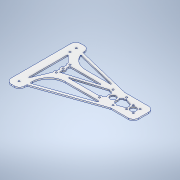
# Autodesk Inventor part: slidesthing
Saved by Autodesk Inventor 2020 (Build 240168000, 168)
## iProperties
Created: 2020-01-10
Part Number: slidesthing
Material: Aluminum 6061
Document SubType Name: Modeling
Designer: xj82b
Density: 2.7 g/cm^3
Appearance: Aluminum - Flat
Mass: 257.407 g
Surface Area: 278.616 cm^2
Volume: 36.001 cm^3
Author: xj82b
Autodesk Inventor part; units mm, degrees
ref_plane "YZ Plane" through (0, 0, 0) normal (1, 0, 0) x (0, 1, 0)
ref_plane "XZ Plane" through (0, 0, 0) normal (0, 1, 0) x (-1, 0, 0)
ref_plane "XY Plane" through (0, 0, 0) normal (0, 0, 1) x (1, 0, 0)
sketch "Sketch1" plane through (0, 0, 0) normal (0, 1, 0) x (-1, 0, 0)
  line L0 (0, 0) -> (0, -286.0722)
  line L1 (0, -286.0722) -> (-32, -286.0722)
  line L2 (-32, -286.0722) -> (-32, -238.0722)
  line L3 (-32, -238.0722) -> (-232, -238.0722)
  line L4 (-232, -238.0722) -> (-232, -190.0722)
  line L5 (-232, -190.0722) -> (-32, -190.0722)
  circle A0 centre (-16, -271.0722) radius 2
  circle A1 centre (-16, -256.0722) radius 2
  circle A2 centre (-16, -136.0722) radius 2
  circle A3 centre (-208, -214.0722) radius 7
  circle A4 centre (-160, -214.0722) radius 7
  circle A5 centre (-42, -230.0722) radius 2
  circle A6 centre (-144, -230.0722) radius 2
  circle A7 centre (-144, -198.0722) radius 2
  circle A8 centre (-176, -198.0722) radius 2
  circle A9 centre (-176, -230.0722) radius 2
  circle A10 centre (-200, -222.0722) radius 2
  circle A11 centre (-216, -222.0722) radius 2
  circle A12 centre (-216, -206.0722) radius 2
  circle A13 centre (-200, -206.0722) radius 2
  circle A14 centre (-42, -214.0722) radius 2
  line L6 (-32, -121.0722) -> (0, -121.0722)
  line L7 (-32, -190.0722) -> (-32, -121.0722)
  point P0 (-32, 0)
  point P1 (-16, -286.0722)
  point P2 (-232, -214.0722)
  dimension "d1" = 32
  dimension "d2" = 48
  dimension "d3" = 48
  dimension "d4" = 4
  dimension "d5" = 4
  dimension "d6" = 4
  dimension "d9" = 150
  dimension "d10" = 15
  dimension "d11" = 30
  dimension "d14" = 216
  dimension "d15" = 14
  dimension "d16" = 14
  dimension "d17" = 24
  dimension "d18" = 48
  dimension "d21" = 4
  dimension "d22" = 8
  dimension "d23" = 42
  dimension "d24" = 4
  dimension "d25" = 4
  dimension "d26" = 4
  dimension "d27" = 4
  dimension "d28" = 32
  dimension "d29" = 32
  dimension "d30" = 16
  dimension "d31" = 16
  dimension "d32" = 4
  dimension "d33" = 4
  dimension "d34" = 4
  dimension "d35" = 4
  dimension "d36" = 16
  dimension "d37" = 16
  dimension "d38" = 8
  dimension "d39" = 8
  dimension "d55" = 4
  dimension "d56" = 16
  dimension "d64" = 15
  dimension "d65" = 69
  constraints: 16 end point, 15 centre point, 7 vertical alignment, 6 horizontal alignment, 4 perpendicular, 3 point on line, 2 midpoint, 1 horizontal, 1 parallel, 1 vertical
  measures "d1" distance of L0.end L1.end
  measures "d2" distance of L1.end L2.end
  measures "d3" distance of L3.end L4.end
  measures "d4" diameter of A0
  measures "d5" diameter of A1
  measures "d6" diameter of A2
  measures "d9" distance from line of L1 A2.centre
  measures "d10" distance from line of L1 A0.centre
  measures "d11" distance from line of A1.centre L1
  measures "d14" distance from line of A1.centre L4
  measures "d15" diameter of A3
  measures "d16" diameter of A4
  measures "d17" distance from line of L4 A3.centre
  measures "d18" distance of A3.centre A4.centre
  measures "d21" diameter of A5
  measures "d22" distance from line of L3 A5.centre
  measures "d23" distance from line of L0 A5.centre
  measures "d24" diameter of A6
  measures "d25" diameter of A7
  measures "d26" diameter of A8
  measures "d27" diameter of A9
  measures "d28" distance of A9.centre A6.centre
  measures "d29" distance of A7.centre A6.centre
  measures "d30" horizontal distance of A4.centre A6.centre
  measures "d31" horizontal distance of A4.centre A6.centre
  measures "d32" diameter of A10
  measures "d33" diameter of A11
  measures "d34" diameter of A12
  measures "d35" diameter of A13
  measures "d36" distance of A11.centre A10.centre
  measures "d37" distance of A12.centre A11.centre
  measures "d38" horizontal distance of A3.centre A11.centre
  measures "d39" horizontal distance of A3.centre A11.centre
  measures "d55" diameter of A14
  measures "d56" distance of A14.centre A5.centre
  measures "d64" distance from line of A2.centre L6
  measures "d65" distance of L5.end L6.start
extrude "Extrusion1" add sketch "Sketch1" along normal blind 3.175
fillet "Fillet1" radius 12 6 edges at (232, 1.5875, -190.0722) (232, 1.5875, -238.0722) (32, 1.5875, -286.0722) (0, 1.5875, -286.0722) (32, 1.5875, -121.0722) (0, 1.5875, -121.0722)
fillet "Fillet2" radius 39 2 edges at (32, 1.5875, -190.0722) (32, 1.5875, -238.0722)
sketch "Sketch2" plane through (0, 3.175, 0) normal (0, 1, 0) x (1, 0, 0)
  circle A0 centre (16, 271.0722) radius 2 construction
  circle A1 centre (16, 271.0722) radius 3 construction
  circle A2 centre (16, 256.0722) radius 3 construction
  circle A3 centre (16, 256.0722) radius 2 construction
  circle A4 centre (42, 230.0722) radius 2 construction
  arc A5 (39.8787, 227.9509) -> (39.1086, 230.872) centre (42, 230.0722) ccw construction
  circle A6 centre (16, 136.0722) radius 2 construction
  circle A7 centre (16, 136.0722) radius 3 construction
  circle A8 centre (144, 230.0722) radius 2 construction
  circle A9 centre (144, 230.0722) radius 3 construction
  circle A10 centre (176, 230.0722) radius 2 construction
  circle A11 centre (176, 230.0722) radius 3 construction
  circle A12 centre (176, 198.0722) radius 2 construction
  circle A13 centre (176, 198.0722) radius 3 construction
  circle A14 centre (144, 198.0722) radius 2 construction
  circle A15 centre (144, 198.0722) radius 3 construction
  circle A16 centre (216, 222.0722) radius 2 construction
  circle A17 centre (216, 222.0722) radius 3 construction
  circle A18 centre (216, 206.0722) radius 2 construction
  circle A19 centre (216, 206.0722) radius 3 construction
  circle A20 centre (200, 206.0722) radius 2 construction
  circle A21 centre (200, 206.0722) radius 3 construction
  circle A22 centre (16, 136.0722) radius 2 construction
  circle A23 centre (176, 230.0722) radius 2 construction
  circle A24 centre (200, 222.0722) radius 3 construction
  circle A25 centre (200, 222.0722) radius 2 construction
  circle A26 centre (200, 206.0722) radius 2 construction
  circle A27 centre (216, 206.0722) radius 2 construction
  circle A28 centre (216, 222.0722) radius 2 construction
  line L0 (13, 136.0722) -> (13, 256.0722)
  line L1 (44.1213, 232.1935) -> (18.1213, 258.1935)
  line L2 (19, 256.0722) -> (19, 135.5292)
  line L3 (39.8787, 227.9509) -> (13.8787, 253.9509)
  circle A29 centre (16, 256.0722) radius 6
  circle A30 centre (42, 230.0722) radius 6
  circle A31 centre (16, 136.0722) radius 6
  circle A32 centre (42, 214.0722) radius 3 construction
  circle A33 centre (42, 214.0722) radius 2 construction
  circle A34 centre (42, 214.0722) radius 6
  line L4 (39, 214.0722) -> (39, 228.8296)
  line L5 (45, 213.5854) -> (45, 230.0722)
  line L6 (39.6062, 233.0722) -> (144, 233.0722)
  line L7 (147, 230.0722) -> (147, 198.0722)
  line L8 (141, 230.0722) -> (141, 198.0722)
  line L9 (144, 227.0722) -> (42, 227.0722)
  line L10 (143.5351, 195.1085) -> (41.5351, 211.1085)
  line L11 (42.4649, 217.036) -> (144.4649, 201.036)
  circle A35 centre (144, 230.0722) radius 6
  circle A36 centre (144, 198.0722) radius 6
  circle A37 centre (42, 198.0722) radius 2
  circle A38 centre (42, 198.0722) radius 3 construction
  circle A39 centre (42, 198.0722) radius 6
  line L12 (42, 201.0722) -> (144.2339, 201.0722)
  line L13 (42, 195.0722) -> (144, 195.0722)
  line L14 (45, 223.4471) -> (45, 216.6383)
  line L15 (45, 214.0722) -> (45, 198.0722)
  line L16 (39, 198.0722) -> (39, 223.6428)
  line L17 (13.2334, 137.2324) -> (39.2334, 199.2324)
  line L18 (18.7666, 134.912) -> (44.7666, 196.912)
  circle A40 centre (176, 230.0722) radius 6
  circle A41 centre (176, 198.0722) radius 2 projected
  circle A42 centre (176, 198.0722) radius 6
  circle A43 centre (200, 206.0722) radius 6
  circle A44 centre (200, 222.0722) radius 6
  circle A45 centre (216, 222.0722) radius 6
  circle A46 centre (216, 206.0722) radius 6
  line L19 (175.0513, 227.2262) -> (199.0513, 219.2262)
  line L20 (197, 222.0722) -> (197, 206.0722)
  line L21 (199.0513, 208.9183) -> (175.0513, 200.9183)
  line L22 (179, 230.0722) -> (179, 198.0722)
  circle A47 centre (3, 196.0722) radius 3 construction
  line L23 (0, 274.0722) -> (0, 133.0722) construction
  circle A48 centre (160, 214.0722) radius 3 construction
  circle A49 centre (160, 214.0722) radius 7 construction
  line L24 (157.8787, 216.1935) -> (141.8787, 200.1935)
  line L25 (141.8787, 227.9509) -> (157.8787, 211.9509)
  circle A50 centre (160, 214.0722) radius 11
  circle A51 centre (208, 214.0722) radius 3 construction
  circle A52 centre (208, 214.0722) radius 7 construction
  line L26 (197.8787, 219.9509) -> (205.8787, 211.9509)
  line L27 (205.8787, 216.1935) -> (197.8787, 208.1935)
  circle A53 centre (208, 214.0722) radius 11
  line L28 (41.102, 200.9347) -> (143.102, 232.9347)
  line L29 (155.4834, 230.5307) -> (160.4569, 232.091)
  line L30 (144.898, 227.2098) -> (42.4595, 195.0722)
  line L31 (15.0089, 138.9038) -> (215.0089, 208.9038)
  line L32 (216.9911, 203.2406) -> (16.9911, 133.2406)
  line L33 (16.7139, 273.986) -> (216.7139, 224.986)
  line L34 (215.2861, 219.1584) -> (15.2861, 268.1584)
  circle A54 centre (16, 271.0722) radius 6
  line L35 (178.1213, 227.9509) -> (162.1213, 211.9509)
  line L36 (162.1213, 216.1935) -> (178.1213, 200.1935)
  line L37 (220, 238.0722) -> (70.9117, 238.0722) projected
  line L38 (163.3009, 238.0722) -> (138.0868, 238.0722)
  point P0 (0, 0)
  point P1 (19, 248.8296)
  point P2 (36.2044, 231.6251)
  point P3 (39, 219.2684)
  point P4 (39, 224.8761)
  point P5 (141, 224.8761)
  point P6 (138.8038, 227.0722)
  point P7 (47.1962, 227.0722)
  point P8 (45, 224.8761)
  point P9 (45, 219.2684)
  point P10 (47.5983, 216.2307)
  point P11 (141, 201.5795)
  point P12 (45, 210.5649)
  point P13 (45, 203.2684)
  point P14 (47.1962, 201.0722)
  point P15 (105.5161, 201.0722)
  point P16 (45, 208.8761)
  point P17 (46.6685, 210.3032)
  point P18 (139.3315, 201.8412)
  point P19 (141, 203.2684)
  point P20 (19, 150.9835)
  point P21 (37.2239, 194.4405)
  point P22 (39, 203.2684)
  point P23 (39, 208.8761)
  point P24 (179, 224.8761)
  point P25 (179, 203.2684)
  point P26 (179.9808, 202.5614)
  point P27 (194.1218, 207.2751)
  point P28 (197, 211.2684)
  point P29 (197, 216.8761)
  point P30 (194.1218, 220.8693)
  point P31 (179.9808, 225.583)
  point P32 (0, 12)
  point P33 (13, 196.0722)
  point P34 (150.3954, 208.7102)
  point P35 (150.3954, 219.4342)
  point P36 (145.5529, 224.2767)
  point P37 (145.5529, 203.8678)
  point P38 (0, 121.0722)
  point P39 (197, 214.0722)
  point P40 (197.3195, 216.7042)
  point P41 (197.3195, 211.4402)
  point P42 (168.1087, 206.6392)
  point P43 (168.1087, 221.5052)
  point P44 (45, 201.0722)
  point P45 (45, 216.6383)
  point P46 (45, 227.0722)
  point P47 (141, 227.0722)
  point P48 (179, 225.9099)
  point P49 (179, 202.2345)
  point P50 (197, 208.2345)
  point P51 (197, 219.9099)
  point P52 (205.368, 224.7527)
  point P53 (205.368, 203.3917)
  point P54 (138.8038, 201.0722)
  point P55 (46.0599, 202.4901)
  point P56 (124.4155, 227.0722)
  point P57 (139.9401, 225.6544)
  point P58 (61.5845, 201.0722)
  point P59 (21.8955, 134.9572)
  point P60 (212.0866, 201.5241)
  point P61 (210.632, 203.3917)
  point P62 (195.5189, 202.0823)
  point P63 (21.3749, 141.1319)
  point P64 (20.7761, 139.7039)
  point P65 (21.7608, 272.7495)
  point P66 (20.333, 266.9219)
  point P67 (170.0027, 230.2528)
  point P68 (181.4016, 227.4601)
  point P69 (194.4175, 224.2712)
  point P70 (210.632, 224.7527)
  point P71 (211.667, 226.2225)
  point P72 (180.6925, 233.8113)
  point P73 (201.0952, 222.6352)
  point P74 (205.9668, 221.4416)
  point P75 (210.2392, 220.3949)
  point P76 (173.5673, 235.5569)
  point P77 (218.6805, 216.7042)
  point P78 (169.6046, 208.7102)
  point P79 (174.4471, 203.8678)
  point P80 (174.4471, 224.2767)
  point P81 (169.6046, 219.4342)
  dimension "d48" = 6
  dimension "d52" = 12
  dimension "d53" = 12
  dimension "d54" = 12
  dimension "d59" = 4
  dimension "d60" = 16
  dimension "d63" = 22
  dimension "d66" = 22
  constraints: 74 end point, 52 tangent, 48 point on circle, 32 centre point, 28 coincident, 23 equal radius, 10 concentric, 9 point on line, 8 vertical, 4 horizontal, 1 horizontal alignment, 1 midpoint, 1 vertical alignment, 31 other
  measures "d48" diameter of A1
  measures "d52" diameter of A29
  measures "d53" diameter of A30
  measures "d54" diameter of A31
  measures "d59" diameter of A37
  measures "d60" distance of A37.centre A32.centre
  measures "d63" diameter of A50
  measures "d66" diameter of A53
extrude "Extrusion3" add sketch "Sketch2" against normal blind 3.175 contours A31 L18 L31 A42 A43 A53 A46 L32 | L31 A42
fillet "Fillet13" radius 2 4 edges at (161.2044, 1.5875, -190.0722) (32, 1.5875, -144.8507) (32, 1.5875, -138.4938) (179.367, 1.5875, -190.0722)
extrude "Extrusion4" cut sketch "Sketch2" against normal through all contours L2 L3 A30 L4 A34 L16 A39 L17 | L15 A34 L10 L28 A39 | A30 L9 L28 L11 A34 L5 | L36 A50 L35 A40 L22 A42 | L21 A42 L22 A40 L19 A44 L20 A43 | L10 A34 L11 L28 | L30 L10 L12 | L20 A53 A43 | L24 L7 L25 A50 | L30 L11 A36 L12 L10 | L20 A44 A53 | L7 L24 A36 L8 A35 L25 | A35 L8 A36 L11 L30 | A37
extrude "Extrusion5" add sketch "Sketch2" against normal blind 3.175 contours L34 A54 L33 L37
fillet "Fillet14" radius 1 6 edges at (34.3544, 1.5875, -263.4866) (138.0868, 1.5875, -238.0722) (124.4155, 1.5875, -227.0722) (61.5845, 1.5875, -201.0722) (19, 1.5875, -248.8296) (19, 1.5875, -150.9835)
body "Solid1"
